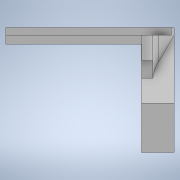
# Autodesk Inventor part: Pi3B_spacer_R_switch2
Saved by Autodesk Inventor 2022 (Build 260153000, 153)
## iProperties
Created: 2023-01-27
Part Number: Pi3B_spacer_R_switch2
Material: Generic
Document SubType Name: Modeling
Designer: scott
Density: 1 g/cm^3
Appearance: Default
Author: scott
Autodesk Inventor part; units mm, degrees
ref_plane "YZ Plane" through (0, 0, 0) normal (1, 0, 0) x (0, 1, 0)
ref_plane "XZ Plane" through (0, 0, 0) normal (0, 1, 0) x (-1, 0, 0)
ref_plane "XY Plane" through (0, 0, 0) normal (0, 0, 1) x (1, 0, 0)
sketch "Sketch1" plane through (0, 0, 0) normal (0, 1, 0) x (-1, 0, 0)
  line L0 (0, 0) -> (21.6, 0)
  line L1 (21.6, 0) -> (21.6, 17)
  line L2 (21.6, 17) -> (0, 17)
  line L3 (0, 17) -> (0, 0)
  line L4 (6.1, 13) -> (3, 13)
  line L5 (3, 13) -> (3, 0)
  line L6 (3, 0) -> (6.1, 0)
  line L7 (6.1, 0) -> (6.1, 13)
  line L8 (21.6, 17) -> (9.1, 17)
  line L9 (9.1, 17) -> (9.1, 0)
  line L10 (9.1, 0) -> (21.6, 0)
  line L11 (21.6, 0) -> (21.6, 17)
  line L12 (9.1, 17) -> (21.6, 6.2)
  point P0 (21.6, 6.2)
  point P1 (9.1, 17)
  dimension "d1" = 17
  dimension "d2" = 3.1
  dimension "d3" = 3
  dimension "d4" = 3
  dimension "d5" = 6.2
  dimension "d17" = 13
  dimension "d18" = 12.5
  constraints: 26 end point, 6 parallel, 3 horizontal, 3 perpendicular, 3 point on line
  measures "d1" distance of L1.end L0.end
  measures "d2" distance between parallel lines of L5 L7
  measures "d3" distance between parallel lines of L3 L5
  measures "d4" distance between parallel lines of L7 L9
  measures "d5" distance from line of L0 L12.end
  measures "d17" distance between parallel lines of L0 L4
  measures "d18" distance between parallel lines of L9 L1
extrude "Extrusion1" add sketch "Sketch1" along normal blind 6 contours L3 L2 L9 L0 L7 L4 L5 | L12 L1 L0 L9
sketch "Sketch2" plane through (-21.6, 0, 0) normal (-1, 0, 0) x (0, 0, 1)
  circle A0 centre (3.1, 3) radius 3
  line L0 (0, 0) -> (13, 0) projected
  line L1 (0, 0) -> (0, 6) projected
  line L2 (17, 6) -> (0, 6) projected
  line L3 (0, 0) -> (6.2302, 0)
  line L4 (6.2302, 0) -> (6.2302, 6)
  line L5 (6.2302, 6) -> (0, 6)
  line L6 (0, 6) -> (0, 0)
  circle A1 centre (3.1, 3) radius 1
  point P0 (3.1, 6)
  point P1 (3.1, 0)
  dimension "d8" = 3.1
  dimension "d9" = 2
  constraints: 8 end point, 2 centre point, 2 parallel, 1 coincident, 1 horizontal, 1 perpendicular, 1 point on line, 1 tangent
  measures "d8" distance from line of L1 A0.centre
  measures "d9" diameter of A1
extrude "Extrusion2" cut sketch "Sketch2" against normal up to surface (18.6 mm away) contours A0 L0 L1 L2 | A1
sketch "Sketch3" plane through (0, 6, 0) normal (0, 1, 0) x (1, 0, 0)
  line L0 (-3, 0) -> (-3, -13) projected
  line L1 (0, 0) -> (-3, 0) projected
  line L2 (-3, -9) -> (0, -9)
  line L3 (0, -9) -> (0, 0)
  line L4 (0, 0) -> (-3, 0)
  line L5 (-3, 0) -> (-3, -9)
  line L6 (-3, -13) -> (-6.1, -13) projected
  line L7 (-9.1, -17) -> (0, -17) projected
  dimension "d13" = 8
  constraints: 8 end point, 2 parallel, 1 horizontal, 1 perpendicular, 1 point on line
  measures "d13" distance between parallel lines of L7 L2
extrude "Extrusion3" cut sketch "Sketch3" against normal blind 10
sketch "Sketch4" plane through (-21.6, 0, 6.2) normal (-1, 0, 0) x (0, 0, 1)
  line L0 (-2.18, -25) -> (8.82, -25)
  line L1 (8.82, -25) -> (8.82, 0)
  line L2 (8.82, 0) -> (-2.18, 0)
  line L3 (-2.18, 0) -> (-2.18, -25)
  circle A0 centre (-3.1, 3) radius 1 projected
  line L4 (0, 0) -> (10.8, 0) projected
  line L5 (0, 0) -> (0, 6) projected
  line L6 (8.82, 0) -> (0, 6)
  circle A1 centre (3.32, -22) radius 1
  circle A2 centre (3.32, -3) radius 1
  line L7 (0.82, -17.5) -> (5.82, -17.5)
  line L8 (5.82, -17.5) -> (5.82, -7.5)
  line L9 (5.82, -7.5) -> (0.82, -7.5)
  line L10 (0.82, -7.5) -> (0.82, -17.5)
  point P0 (-6.2, 0)
  dimension "d19" = 0.92
  dimension "d20" = 0
  dimension "d21" = 25
  dimension "d22" = 11
  dimension "d23" = 5.5
  dimension "d24" = 5.5
  dimension "d25" = 5
  dimension "d26" = 10
  dimension "d27" = 7.5
  dimension "d28" = 3
  dimension "d29" = 2
  dimension "d30" = 2
  dimension "d51" = 19
  dimension "d52" = 3
  constraints: 18 end point, 4 parallel, 2 centre point, 2 horizontal, 2 perpendicular
  measures "d19" distance from line of L3 A0.centre
  measures "d20" distance between parallel lines of L4 L2
  measures "d21" distance of L2.end L0.start
  measures "d22" distance of L0.start L0.end
  measures "d23" distance from line of L3 A1.centre
  measures "d24" distance from line of L3 A2.centre
  measures "d25" distance between parallel lines of L8 L10
  measures "d26" distance between parallel lines of L9 L7
  measures "d27" distance between parallel lines of L0 L7
  measures "d28" distance between parallel lines of L3 L10
  measures "d29" diameter of A1
  measures "d30" diameter of A2
  measures "d51" distance of A2.centre A1.centre
  measures "d52" distance from line of L0 A1.centre
extrude "Extrusion4" add sketch "Sketch4" against normal blind 1.7 contours L3 L2 L1 L0 | L2 L5 L6
sketch "Sketch6" plane through (0, 0, 0) normal (0, -1, 0) x (1, 0, 0)
  line L0 (-19.9, 15.02) -> (-19.9, 4.02) projected
  line L1 (-19.9, 4.02) -> (-7.9, 4.02)
  line L2 (-7.9, 4.02) -> (-7.9, 15.02)
  line L3 (-7.9, 15.02) -> (-19.9, 15.02)
  line L4 (-19.9, 15.02) -> (-19.9, 4.02)
  line L5 (-12.9, 4.02) -> (-10.3572, 4.02)
  line L6 (-10.3572, 4.02) -> (-10.3572, 15.02)
  line L7 (-10.3572, 15.02) -> (-12.9, 15.02)
  line L8 (-12.9, 15.02) -> (-12.9, 4.02)
  line L9 (-12.9, 15.02) -> (-16.9, 15.02)
  line L10 (-16.9, 15.02) -> (-16.9, 13.02)
  line L11 (-16.9, 13.02) -> (-12.9, 13.02)
  line L12 (-12.9, 13.02) -> (-12.9, 15.02)
  line L13 (-21.6, 15.02) -> (-21.6, 6.2) projected
  line L14 (-19.9, 4.02) -> (-21.6, 4.02)
  line L15 (-21.6, 4.02) -> (-21.6, 15.02)
  line L16 (-21.6, 15.02) -> (-19.9, 15.02)
  line L17 (-19.9, 15.02) -> (-19.9, 4.02)
  point P0 (0, 0)
  dimension "d33" = 12
  dimension "d34" = 7
  dimension "d35" = 4
  dimension "d36" = 2
  constraints: 32 end point, 8 parallel, 4 horizontal, 4 perpendicular, 2 point on line
  measures "d33" distance of L3.end L2.end
  measures "d34" distance between parallel lines of L0 L8
  measures "d35" distance of L11.end L10.end
  measures "d36" distance of L10.end L9.end
extrude "Extrusion5" add sketch "Sketch6" against normal blind 2 contours L3 L10 L11 L8 L1 L0 | L0 L14 L15 L13 L16
sketch "Sketch7" plane through (-21.6, 3, 3.1) normal (-1, 0, 0) x (0, 0, 1)
  line L0 (8.98, -1) -> (3.1, 3) projected
  line L1 (8.98, -1) -> (3.1, -1)
  line L2 (3.1, -1) -> (3.1, 3)
  line L3 (3.1, 3) -> (8.98, 3)
  line L4 (8.98, 3) -> (8.98, -1)
  line L5 (0, 3) -> (3.1, 3) projected
  line L6 (3.1, 3) -> (8.98, -1)
  point P0 (-3.1, -3)
  constraints: 10 end point, 2 parallel, 1 horizontal, 1 perpendicular
extrude "Extrusion6" add sketch "Sketch7" against normal blind 9 contours L1 L2 L0
sketch "Sketch8" plane through (-21.6, 3, 3.1) normal (-1, 0, 0) x (0, 0, 1)
  line L0 (-9.7709, -24.08) -> (2.92, -24.08)
  line L1 (2.92, -24.08) -> (2.92, 6.3077)
  line L2 (2.92, 6.3077) -> (-9.7709, 6.3077)
  line L3 (-9.7709, 6.3077) -> (-9.7709, -24.08)
  line L4 (11.92, -28) -> (11.92, -1) projected
  line L5 (0.92, -28) -> (11.92, -28) projected
  line L6 (0.92, -3) -> (0.92, -28) projected
  line L7 (3.1, 3) -> (8.98, -1) projected
  line L8 (0.92, -28) -> (3.92, -28)
  line L9 (3.92, -28) -> (3.92, 2.4422)
  line L10 (3.92, 2.4422) -> (0.92, 2.4422)
  line L11 (0.92, 2.4422) -> (0.92, -28)
  line L12 (3.92, -20.5) -> (3.92, -10.5) projected
  line L13 (2.92, 2.4422) -> (2.92, 3)
  line L14 (3.1, 3) -> (13.9, 3) projected
  line L15 (2.92, 2.4422) -> (3.92, 2.4422)
  line L16 (3.92, 2.4422) -> (3.92, 3)
  line L17 (3.92, 3) -> (2.92, 3)
  line L18 (2.92, 3) -> (2.92, 2.4422)
  line L19 (3.92, 2.4422) -> (3.1, 3)
  point P0 (-3.1, -3)
  point P1 (0.92, -24.08)
  point P2 (3.92, -28)
  point P3 (2.92, 3)
  dimension "d41" = 9
  dimension "d42" = 3.92
  dimension "d43" = 10.691
  dimension "d44" = 0
  dimension "d45" = 0
  constraints: 28 end point, 7 point on line, 6 parallel, 3 horizontal, 3 perpendicular, 1 collinear
  measures "d41" distance between parallel lines of L1 L4
  measures "d42" distance between parallel lines of L5 L0
  measures "d43" distance between parallel lines of L6 L3
  measures "d44" distance between parallel lines of L12 L9
  measures "d45" distance between parallel lines of L5 L8
extrude "Extrusion7" add sketch "Sketch8" along normal blind 1.4 contours L0 L1 L10 L9 L5 L6 | L1 L17 L7 L10
fillet "Fillet1" radius 2 1 edges at (-22.3, -21.08, 6.02)
fillet "Fillet2" radius 6 1 edges at (-18.1972, 2, 12.08)
fillet "Fillet3" radius 2 1 edges at (-19.25, 2, 15.02)
equation "\"d23\" = 0.5 * d22"
equation "\"d24\" = 0.5 * d22"
equation "\"d27\" = -0.5 * d26 + 0.5 * d21"
equation "\"d28\" = -0.5 * d25 + 0.5 * d22"
equation "\"d52\" = -0.5 * d51 + 0.5 * d21"
body "Solid1"
